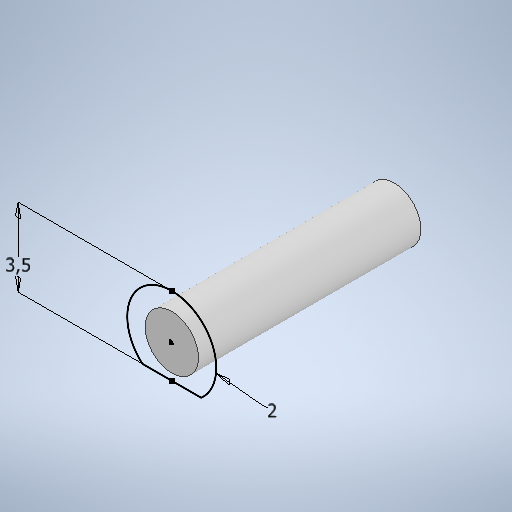
# Autodesk Inventor part: 13042026-08
Saved by Autodesk Inventor 2025.2 (Build 292293000, 293)
## iProperties
Created: 2026-05-06
Part Number: 13042026-08
Material: Generic
Document SubType Name: Modeling
Designer: Oski
Density: 1 g/cm^3
Appearance: Default
Author: Oski
Autodesk Inventor part; units mm, degrees
ref_plane "YZ Plane" through (0, 0, 0) normal (1, 0, 0) x (0, 1, 0)
ref_plane "XZ Plane" through (0, 0, 0) normal (0, 1, 0) x (-1, 0, 0)
ref_plane "XY Plane" through (0, 0, 0) normal (0, 0, 1) x (1, 0, 0)
sketch "Sketch1" plane through (0, 0, 0) normal (0, 0, 1) x (1, 0, 0)
  circle A0 centre (0, 0) radius 1.2
  dimension "d0" = 2.4
  constraints: 1 centre point, 1 coincident
  measures "d0" diameter of A0
extrude "Extrusion1" add sketch "Sketch1" along normal mid plane 10
sketch "Sketch2" plane through (0, 0, 5) normal (0, 0, 1) x (1, 0, 0)
  arc A0 (1.3229, -1.5) -> (-1.3229, -1.5) centre (0, 0) ccw
  line L0 (-1.3229, -1.5) -> (1.3229, -1.5)
  point P0 (0, -1.5)
  point P1 (0, 2)
  dimension "d3" = 3.5
  dimension "d4" = 2
  constraints: 3 point on circle, 2 end point, 1 centre point, 1 coincident, 1 horizontal, 1 midpoint
  measures "d3" distance of point (0, -1.5) point (0, 2)
  measures "d4" radius of A0
body "Solid1"
